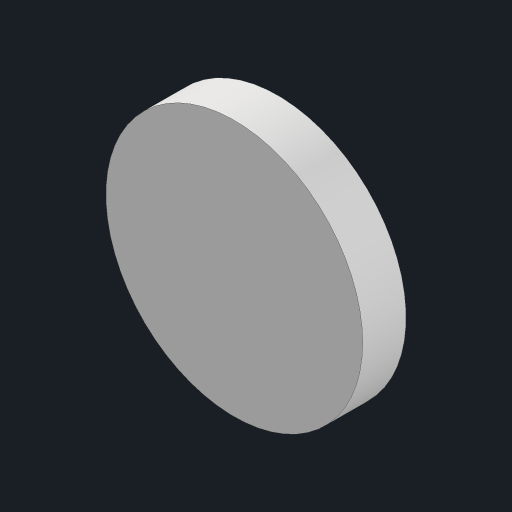
# Autodesk Inventor part: dol_do_wylania
Saved by Autodesk Inventor 2023 (Build 270158000, 158)
## iProperties
Created: 2024-06-30
Part Number: dol_do_wylania
Material: Generic
Document SubType Name: Modeling
Designer: szymo
Density: 1 g/cm^3
Appearance: Default
Mass: 14.5871 g
Surface Area: 73.5269 cm^2
Volume: 14.5871 cm^3
Author: szymo
Autodesk Inventor part; units mm, degrees
ref_plane "YZ Plane" through (0, 0, 0) normal (1, 0, 0) x (0, 1, 0)
ref_plane "XZ Plane" through (0, 0, 0) normal (0, 1, 0) x (-1, 0, 0)
ref_plane "Work Plane1" through (-18.5, -18.5, -2) normal (0, 0, -1) x (0, 1, 0)
sketch "Sketch1" plane through (0, 0, 0) normal (0, 0, 1) x (1, 0, 0)
  circle A0 centre (0, 0) radius 22.5
  circle A1 centre (0, 0) radius 12.7 projected
  dimension "d0" = 45
  constraints: 1 centre point, 1 coincident
  measures "d0" diameter of A0
extrude "Extrusion1" add sketch "Sketch1" against normal up to surface (2 mm away) contours A1
sketch "Sketch2" plane through (0, 0, 0) normal (0, 0, 1) x (1, 0, 0)
  circle A0 centre (0, 0) radius 22.6
  dimension "d3" = 45.2
  constraints: 1 centre point, 1 coincident
  measures "d3" diameter of A0
extrude "Extrusion2" add sketch "Sketch2" along normal blind 7
sketch "Sketch3" plane through (0, 0, 7) normal (0, 0, -1) x (-1, 0, 0)
  circle A0 centre (0, 0) radius 12.7
  line L0 (12.7, 0) -> (-12.7, 0)
  circle A1 centre (10.7, 0) radius 2
  circle A2 centre (-10.7, 0) radius 2
  line L1 (7.4668, 0) -> (9.0834, 2.8)
  line L2 (9.0834, 2.8) -> (12.3166, 2.8)
  line L3 (12.3166, 2.8) -> (13.9332, 0)
  line L4 (13.9332, 0) -> (12.3166, -2.8)
  line L5 (12.3166, -2.8) -> (9.0834, -2.8)
  line L6 (9.0834, -2.8) -> (7.4668, 0)
  line L7 (-7.4668, 0) -> (-9.0834, -2.8)
  line L8 (-9.0834, -2.8) -> (-12.3166, -2.8)
  line L9 (-12.3166, -2.8) -> (-13.9332, 0)
  line L10 (-13.9332, 0) -> (-12.3166, 2.8)
  line L11 (-12.3166, 2.8) -> (-9.0834, 2.8)
  line L12 (-9.0834, 2.8) -> (-7.4668, 0)
  circle A3 centre (0, 0) radius 12.7 projected
  point P0 (0, 0)
  dimension "d6" = 4
  dimension "d7" = 4
  dimension "d8" = 5.6
  dimension "d9" = 5.6
  constraints: 26 end point, 5 coincident, 4 point on line, 3 centre point, 2 midpoint, 2 point on circle, 2 tangent, 1 concentric, 1 horizontal, 26 other
  measures "d6" diameter of A1
  measures "d7" diameter of A2
  measures "d8" distance between parallel lines of L1 L4
  measures "d9" distance from line of L9 L7.start
hole "Hole1" at (-10.7, 0, 7) at (10.7, 0, 7) direction (0, 0, -1) diameter 3.6 end through all countersink diameter 7 countersink angle 90 clearance for "Countersunk Flat Head Screw ISO 2009/7046" size "M3" standard "ISO"
sketch "Sketch4" plane through (0, 0, 7) normal (0, 0, 1) x (1, 0, 0)
  circle A0 centre (0, 0) radius 22.6 projected
  circle A1 centre (0, 0) radius 25.15
  circle A2 centre (0, 0) radius 26.65
  dimension "d17" = 50.3
  dimension "d18" = 1.5
  constraints: 2 centre point, 1 coincident
  measures "d17" diameter of A1
  measures "d18" radial gap between concentric circles of A1 A2
extrude "Extrusion3" add sketch "Sketch4" against normal blind 2 contours A0 | A1 | A2
sketch "Sketch5" plane through (0, 0, 5) normal (0, 0, -1) x (-1, 0, 0)
  circle A0 centre (0, 0) radius 25.1
  circle A1 centre (0, 0) radius 26.65 projected
  dimension "d21" = 50.2
  constraints: 1 centre point, 1 coincident
  measures "d21" diameter of A0
extrude "Extrusion4" add sketch "Sketch5" along normal blind 7
fillet "Fillet1" radius 0.6 3 edges at (25.1, 0, -2) (-22.6, 0, 0) (-12.7, 0, -2)
body "Solid1"
